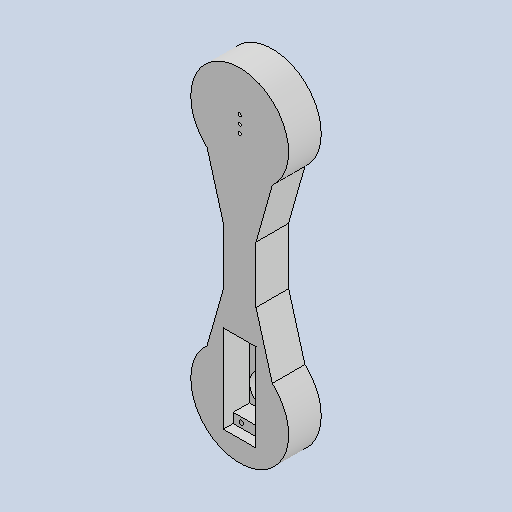
# Autodesk Inventor part: 1stArm
Saved by Autodesk Inventor 2022 (Build 260153000, 153)
## iProperties
Created: 2022-02-11
Part Number: 1stArm
Material: Generic
Document SubType Name: Modeling
Designer: Alexa
Density: 1 g/cm^3
Appearance: Default
Mass: 133.239 g
Surface Area: 290.961 cm^2
Volume: 133.239 cm^3
Author: Alexa
Autodesk Inventor part; units mm, degrees
ref_plane "YZ Plane" through (0, 0, 0) normal (1, 0, 0) x (0, 1, 0)
ref_plane "XZ Plane" through (0, 0, 0) normal (0, 1, 0) x (-1, 0, 0)
ref_plane "XY Plane" through (0, 0, 0) normal (0, 0, 1) x (1, 0, 0)
sketch "Sketch1" plane through (0, 0, 0) normal (0, 0, 1) x (1, 0, 0)
  line L0 (0, 0) -> (40, 0)
  line L1 (40, 0) -> (40, 150)
  line L2 (40, 150) -> (0, 150)
  line L3 (0, 150) -> (0, 0)
  circle A0 centre (20, 0) radius 30
  circle A1 centre (20, 150) radius 30
  point P0 (0, 22.3607)
  point P1 (40, 22.3607)
  point P2 (40, 127.6393)
  point P3 (0, 127.6393)
  dimension "d0" = 40
  dimension "d1" = 150
  dimension "d2" = 60
  dimension "d3" = 60
  constraints: 8 end point, 2 centre point, 2 midpoint, 2 parallel, 1 horizontal, 1 perpendicular
  measures "d0" distance of L2.end L1.end
  measures "d1" distance of L1.end L0.end
  measures "d2" diameter of A0
  measures "d3" diameter of A1
extrude "Extrusion1" add sketch "Sketch1" along normal blind 20
sketch "Sketch2" plane through (0, 0, 20) normal (0, 0, 1) x (1, 0, 0)
  line L0 (10, 0) -> (30, 0)
  line L1 (30, 0) -> (30, -17)
  line L2 (30, -17) -> (10, -17)
  line L3 (10, -17) -> (10, 0)
  line L4 (10, 0) -> (30, 0)
  line L5 (30, 0) -> (30, 36.8)
  line L6 (30, 36.8) -> (10, 36.8)
  line L7 (10, 36.8) -> (10, 0)
  line L8 (10, 36.8) -> (30, 36.8)
  line L9 (30, 36.8) -> (30, 30.8)
  line L10 (30, 30.8) -> (10, 30.8)
  line L11 (10, 30.8) -> (10, 36.8)
  line L12 (10, -17) -> (30, -17)
  line L13 (30, -17) -> (30, -11)
  line L14 (30, -11) -> (10, -11)
  line L15 (10, -11) -> (10, -17)
  line L16 (10, 36.8) -> (30, 36.8)
  line L17 (30, 36.8) -> (30, 33.8)
  line L18 (30, 33.8) -> (10, 33.8)
  line L19 (10, 33.8) -> (10, 36.8)
  line L20 (10, -17) -> (30, -17)
  line L21 (30, -17) -> (30, -14)
  line L22 (30, -14) -> (10, -14)
  line L23 (10, -14) -> (10, -17)
  point P0 (0, 0)
  dimension "d6" = 20
  dimension "d7" = 17
  dimension "d8" = 36.8
  dimension "d9" = 6
  dimension "d10" = 6
  dimension "d11" = 3
  constraints: 48 end point, 12 parallel, 6 horizontal, 6 perpendicular, 3 point on line, 2 midpoint
  measures "d6" distance of L1.end L2.end
  measures "d7" distance of L0.end L1.end
  measures "d8" distance of L5.end L4.end
  measures "d9" distance of L8.end L9.end
  measures "d10" distance of L13.end L12.end
  measures "d11" distance of L16.end L17.end
extrude "Extrusion2" cut sketch "Sketch2" against normal blind 16 contours L7 L10 L5 L0 | L0 L1 L14 L3
sketch "Sketch3" plane through (0, 0, 0) normal (0, 0, -1) x (-1, 0, 0)
  circle A0 centre (-20, 0) radius 10
  point P0 (0, 0)
  dimension "d14" = 20
  constraints: 1 centre point
  measures "d14" diameter of A0
extrude "Extrusion3" cut sketch "Sketch3" against normal blind 69.725
sketch "Sketch4" plane through (0, 0, 20) normal (0, 0, 1) x (1, 0, 0)
  line L0 (30, -11) -> (10, -11)
  line L1 (10, -11) -> (10, -17)
  line L2 (10, -17) -> (30, -17)
  line L3 (30, -17) -> (30, -11)
  line L4 (30, 30.8) -> (30, 0) projected
  line L5 (30, 30.8) -> (10, 30.8)
  line L6 (10, 30.8) -> (10, 36.8)
  line L7 (10, 36.8) -> (30, 36.8)
  line L8 (30, 36.8) -> (30, 30.8)
  line L9 (30, -17) -> (10, -17)
  line L10 (10, -17) -> (10, -14)
  line L11 (10, -14) -> (30, -14)
  line L12 (30, -14) -> (30, -17)
  point P0 (0, 0)
  dimension "d17" = 6
  dimension "d18" = 6
  constraints: 24 end point, 6 parallel, 3 horizontal, 3 perpendicular, 1 midpoint, 1 point on line
  measures "d17" distance of L1.end L0.end
  measures "d18" distance of L5.end L6.end
extrude "Extrusion4" cut sketch "Sketch4" against normal blind 6
sketch "Sketch5" plane through (0, 0, 14) normal (0, 0, 1) x (1, 0, 0)
  line L0 (30, 36.8) -> (30, -17) projected
  line L1 (10, -17) -> (10, 36.8) projected
  line L2 (30, -17) -> (10, -17)
  line L3 (10, -17) -> (10, -14)
  line L4 (10, -14) -> (30, -14)
  line L5 (30, -14) -> (30, -17)
  line L6 (20, -14) -> (15, -14)
  line L7 (15, -14) -> (15, -13.2117)
  line L8 (15, -13.2117) -> (20, -13.2117)
  line L9 (20, -13.2117) -> (20, -14)
  line L10 (20, -14) -> (25, -14)
  line L11 (25, -14) -> (25, -13.2117)
  line L12 (25, -13.2117) -> (20, -13.2117)
  line L13 (20, -13.2117) -> (20, -14)
  circle A0 centre (25, -14) radius 1.35
  circle A1 centre (15, -14) radius 1.35
  line L14 (10, 36.8) -> (30, 36.8) projected
  line L15 (10, 30.8) -> (10, 36.8) projected
  line L16 (30, 36.8) -> (10, 36.8)
  line L17 (10, 36.8) -> (10, 33.8)
  line L18 (10, 33.8) -> (30, 33.8)
  line L19 (30, 33.8) -> (30, 36.8)
  line L20 (20, 33.8) -> (25, 33.8)
  line L21 (25, 33.8) -> (25, 32.7882)
  line L22 (25, 32.7882) -> (20, 32.7882)
  line L23 (20, 32.7882) -> (20, 33.8)
  line L24 (20, 33.8) -> (15, 33.8)
  line L25 (15, 33.8) -> (15, 32.7882)
  line L26 (15, 32.7882) -> (20, 32.7882)
  line L27 (20, 32.7882) -> (20, 33.8)
  circle A2 centre (25, 33.8) radius 1.35
  circle A3 centre (15, 33.8) radius 1.35
  point P0 (0, 0)
  dimension "d21" = 3
  dimension "d22" = 5
  dimension "d23" = 5
  dimension "d24" = 2.7
  dimension "d25" = 2.7
  dimension "d26" = 3
  dimension "d27" = 2.7
  dimension "d28" = 2.7
  constraints: 48 end point, 12 parallel, 6 horizontal, 6 perpendicular, 4 centre point, 4 coincident, 3 midpoint, 3 point on line
  measures "d21" distance of L2.end L3.end
  measures "d22" distance of L7.end L8.end
  measures "d23" distance of L12.end L11.end
  measures "d24" diameter of A0
  measures "d25" diameter of A1
  measures "d26" distance of L17.end L16.end
  measures "d27" diameter of A2
  measures "d28" diameter of A3
extrude "Extrusion5" cut sketch "Sketch5" against normal blind 10 contours A2 L22 L21 L18 | L18 A2 | A0 L4 | L4 L11 L12 A0 | L21 L22 A2 L18 | A3 L18 | L18 L25 L26 A3 | L4 A0 L12 L11 | L18 A3 L26 L25 | A1 L8 L7 L4 | L4 A1 | A1 L4 L7 L8
thread "Thread1" size "M3x0.5" class "6H" standard "ANSI Metric M Profile" full length
thread "Thread2" size "M3x0.5" class "6H" standard "ANSI Metric M Profile" full length
thread "Thread3" size "M3x0.5" class "6H" standard "ANSI Metric M Profile" full length
thread "Thread4" size "M3x0.5" class "6H" standard "ANSI Metric M Profile" full length
sketch "Sketch6" plane through (0, 0, 0) normal (0, 0, -1) x (-1, 0, 0)
  line L0 (0, 0) -> (-20, 0)
  line L1 (-20, 0) -> (-20, 150)
  line L2 (-20, 150) -> (0, 150)
  line L3 (0, 150) -> (0, 0)
  circle A0 centre (-20, 150) radius 10
  circle A1 centre (-25, 150) radius 1
  circle A2 centre (-15, 150) radius 1
  circle A3 centre (-20, 150) radius 1
  dimension "d39" = 20
  dimension "d40" = 150
  dimension "d41" = 20
  dimension "d42" = 2
  dimension "d43" = 2
  dimension "d44" = 2
  constraints: 8 end point, 4 centre point, 2 coincident, 2 parallel, 1 horizontal, 1 perpendicular
  measures "d39" distance of L1.end L2.end
  measures "d40" distance of L0.end L1.end
  measures "d41" diameter of A0
  measures "d42" diameter of A1
  measures "d43" diameter of A2
  measures "d44" diameter of A3
extrude "Extrusion6" cut sketch "Sketch6" against normal blind 39.2125 contours A3 L2 L1 | L1 L2 A3 | A2 L2 | L2 A2 | A1
sketch "Sketch7" plane through (0, 0, 20) normal (0, 0, 1) x (1, 0, 0)
  circle A0 centre (20, 150) radius 10
  point P0 (0, 0)
  dimension "d47" = 20
  constraints: 1 centre point
  measures "d47" diameter of A0
extrude "Extrusion7" cut sketch "Sketch7" against normal blind 16
sketch "Sketch8" plane through (0, 0, 20) normal (0, 0, 1) x (1, 0, 0)
  line L0 (40, 22.3607) -> (40, 127.6393) projected
  line L1 (0, 127.6393) -> (40, 127.6393)
  line L2 (40, 127.6393) -> (40, 22.3607)
  line L3 (40, 22.3607) -> (0, 22.3607)
  line L4 (0, 22.3607) -> (0, 127.6393)
  line L5 (10, 0) -> (10, 30.8) projected
  line L6 (10, 22.3607) -> (30, 22.3607)
  line L7 (30, 22.3607) -> (30, 92.3607)
  line L8 (30, 92.3607) -> (10, 92.3607)
  line L9 (10, 92.3607) -> (10, 22.3607)
  line L10 (10, 127.6393) -> (30, 127.6393)
  line L11 (30, 127.6393) -> (30, 57.6393)
  line L12 (30, 57.6393) -> (10, 57.6393)
  line L13 (10, 57.6393) -> (10, 127.6393)
  line L14 (0, 127.6393) -> (10, 92.3607)
  line L15 (30, 92.3607) -> (40, 127.6393)
  line L16 (0, 127.6393) -> (0, 22.3607) projected
  line L17 (10, 57.6393) -> (0, 22.3607)
  line L18 (30, 57.6393) -> (40, 22.3607)
  point P0 (0, 0)
  dimension "d53" = 20
  dimension "d54" = 70
  dimension "d55" = 70
  constraints: 32 end point, 6 parallel, 5 point on line, 3 horizontal, 3 perpendicular
  measures "d53" distance of L8.end L7.end
  measures "d54" distance of L7.end L6.end
  measures "d55" distance of L10.end L11.end
extrude "Extrusion8" cut sketch "Sketch8" against normal blind 56.675 contours L18 L7 L15 L0 | L17 L4 L14 L9
sketch "Sketch9" plane through (0, 0, 20) normal (0, 0, 1) x (1, 0, 0)
  circle A0 centre (20, 150) radius 10 projected
  circle A1 centre (20, 150) radius 10
  point P0 (0, 0)
  constraints: 1 centre point, 1 coincident
extrude "Extrusion9" add sketch "Sketch9" against normal blind 16
sketch "Sketch10" plane through (0, 0, 0) normal (0, 0, -1) x (-1, 0, 0)
  circle A0 centre (-20, 150) radius 1 projected
  circle A1 centre (-20, 150) radius 10
  point P0 (0, 0)
  dimension "d60" = 20
  constraints: 1 centre point, 1 coincident
  measures "d60" diameter of A1
extrude "Extrusion10" cut sketch "Sketch10" against normal blind 16
sketch "Sketch11" plane through (0, 0, 0) normal (0, 0, -1) x (-1, 0, 0)
  circle A0 centre (-20, 150) radius 1
  point P0 (0, 0)
  constraints: 1 centre point
extrude "Extrusion11" add sketch "Sketch11" against normal blind 20
sketch "Sketch12" plane through (20, 150, 0) normal (0, 0, -1) x (-1, 0, 0)
  circle A0 centre (0, 0) radius 1
  point P0 (20, -150)
  constraints: 1 centre point
extrude "Extrusion12" cut sketch "Sketch12" against normal blind 49.85
sketch "Sketch13" plane through (20, 150, 16) normal (0, 0, -1) x (-1, 0, 0)
  circle A0 centre (0, -5) radius 1
  circle A1 centre (0, 5) radius 1
  point P0 (20, -150)
  dimension "d67" = 2
  dimension "d68" = 2
  constraints: 2 centre point
  measures "d67" diameter of A0
  measures "d68" diameter of A1
extrude "Extrusion13" cut sketch "Sketch13" against normal blind 42.225
chamfer "Chamfer2" distance 12 angle 45 1 edges at (30, 150, 0)
body "Solid1"
